# Autodesk Inventor part: Pushbutton
Saved by Autodesk Inventor 2013 (Build 170138000, 138)
## iProperties
Created: 2013-01-27
Part Number: Pushbutton
Material: Generic
Document SubType Name: Modeling
Designer: davidgitz
Density: 1 g/cm^3
Author: davidgitz
Autodesk Inventor part; units mm, degrees
ref_plane "YZ Plane" through (0, 0, 0) normal (1, 0, 0) x (0, 1, 0)
ref_plane "XZ Plane" through (0, 0, 0) normal (0, 1, 0) x (-1, 0, 0)
ref_plane "XY Plane" through (0, 0, 0) normal (0, 0, 1) x (1, 0, 0)
sketch "FSM2JH, Pushbutton_60" plane through (0, 0, 0) normal (0, 0, 1) x (1, 0, 0)
  line L0 (1.6251, 0.2499) -> (4.3749, 0.2499)
  arc A0 (4.3749, 0.2499) -> (5.125, 1) centre (4.3749, 1) ccw
  line L1 (5.125, 1) -> (5.125, 3.5001)
  arc A1 (5.125, 3.5001) -> (4.3749, 4.2499) centre (4.375, 3.5) ccw
  line L2 (4.3749, 4.2499) -> (1.6251, 4.2499)
  arc A2 (1.6251, 4.2499) -> (0.875, 3.5001) centre (1.625, 3.5) ccw
  line L3 (0.875, 3.5001) -> (0.875, 1)
  arc A3 (0.875, 1) -> (1.6251, 0.2499) centre (1.6251, 1) ccw
  constraints: 8 end point, 8 point on circle, 4 centre point
extrude "Extrusion1" add sketch "FSM2JH, Pushbutton_60" along normal blind 6.35
body "Solid1"
